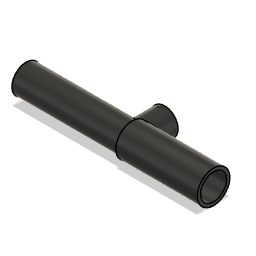
Canon (Autodesk Fusion 360 design; units mm, degrees)
Autodesk Fusion 360 part; units mm, degrees
sketch "Sketch1" plane through (0, 0, 0) normal (0, 0, 1) x (1, 0, 0)
  circle A0 centre (0, 0) radius 16.5
  circle A1 centre (0, 0) radius 15.5
  line L0 (-25, -5) -> (25, -5)
  line L1 (25, -5) -> (25, 5)
  line L2 (25, 5) -> (-25, 5)
  line L3 (-25, 5) -> (-25, -5)
  line L4 (-25, -5) -> (25, 5) construction
  line L5 (25, -5) -> (-25, 5) construction
  line L6 (-5, 25) -> (5, 25)
  line L7 (5, 25) -> (5, -25)
  line L8 (5, -25) -> (-5, -25)
  line L9 (-5, -25) -> (-5, 25)
  line L10 (-5, 25) -> (5, -25) construction
  line L11 (5, 25) -> (-5, -25) construction
  circle A2 centre (0, 4) radius 1
  circle A3 centre (0, -4) radius 1
  circle A4 centre (-3, 0) radius 1
  circle A5 centre (3, 0) radius 1
  dimension "d1" = 33
  dimension "d15" = 31
  dimension "d18" = 50
  dimension "d19" = 10
  dimension "d20" = 10
  dimension "d21" = 50
  dimension "d22" = 2
  dimension "d23" = 2
  dimension "d25" = 2
  dimension "d26" = 4
  dimension "d27" = 8
  dimension "d28" = 2
  dimension "d29" = 3
  dimension "d30" = 6
  constraint coincident A0.centre A1.centre
  constraint horizontal L0
  constraint perpendicular L0 L1
  constraint parallel L0 L2
  constraint parallel L1 L3
  constraint coincident L4 A0.centre
  constraint coincident L5 A0.centre
  constraint horizontal L6
  constraint perpendicular L6 L7
  constraint parallel L6 L8
  constraint parallel L7 L9
  constraint coincident L10 A0.centre
  constraint coincident L11 A0.centre
  measures "d1" diameter of A0
  measures "d15" diameter of A1
  measures "d18" distance of L1.end L2.end
  measures "d19" distance of L0.end L1.end
  measures "d20" distance of L7.end L8.end
  measures "d21" distance of L6.end L7.end
  measures "d22" diameter of A2
  measures "d23" diameter of A3
  measures "d25" diameter of A4
  measures "d26" distance of A0.centre A3.centre
  measures "d27" distance of A2.centre A3.centre
  measures "d28" diameter of A5
  measures "d29" distance of A0.centre A5.centre
  measures "d30" distance of A4.centre A5.centre
extrude "Extrude1" add sketch "Sketch1" along normal blind 37 contours A0 A1 L0 L2 | A0 A1 L2 L7 | A0 A1 L0 L7 | A0 A1 L7 L9 | A1 L2 L7 | A1 L0 L2 L7 | A0 A1 L7 L9 | A1 L0 L7 | A0 A1 L2 L9 | A1 L2 L7 L9 | A2 | A3 | L0 L2 L7 L9 | A0 A1 L0 L9 | A1 L0 L7 L9 | A0 A1 L0 L2 | A1 L2 L9 | A1 L0 L9 | A1 L0 L2 L9 | A4 | A5
sketch "Sketch2" plane through (0, 0, 0) normal (1, 0, 0) x (0, 0, -1)
  circle A0 centre (-39.9957, 0.4126) radius 20
  circle A1 centre (-39.9957, 0.4126) radius 17.5
  circle A2 centre (-39.9957, 0.4126) radius 16
  dimension "d4" = 40
  dimension "d7" = 35
  dimension "d10" = 32
  constraint concentric A0 A1
  constraint concentric A1 A2
  measures "d4" diameter of A0
  measures "d7" diameter of A1
  measures "d10" diameter of A2
extrude "Extrude2" add sketch "Sketch2" along normal blind 100 contours A0 | A1 | A2
extrude "Extrude3" add sketch "Sketch2" against normal blind 130 contours A1 | A2
extrude "Extrude4" cut sketch "Sketch2" along normal blind 140 and the other way blind 90 contours A2
extrude "Extrude5" cut sketch "Sketch1" along normal blind 40 contours A1 L2 L7 | A1 L0 L2 L7 | A1 L0 L7 | A1 L2 L7 L9 | A2 | A3 | L0 L2 L7 L9 | A1 L0 L7 L9 | A1 L2 L9 | A1 L0 L9 | A1 L0 L2 L9 | A4 | A5
extrude "Extrude6" add sketch "Sketch1" along normal blind 2 from surface at 3 contours A1 L0 L2 L7 | A1 L2 L7 L9 | L0 L2 L7 L9 | A1 L0 L7 L9 | A1 L0 L2 L9
